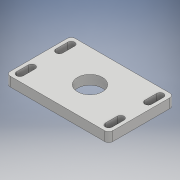
# Autodesk Inventor part: belt tensioner
Saved by Autodesk Inventor 2017 (Build 210142000, 142)
## iProperties
Created: 2018-04-16
Part Number: belt tensioner
Material: Generic
Document SubType Name: Modeling
Designer: RKL
Density: 1 g/cm^3
Appearance: Default
Author: RKL
Autodesk Inventor part; units mm, degrees
ref_plane "YZ Plane" through (0, 0, 0) normal (1, 0, 0) x (0, 1, 0)
ref_plane "XZ Plane" through (0, 0, 0) normal (0, 1, 0) x (-1, 0, 0)
ref_plane "XY Plane" through (0, 0, 0) normal (0, 0, 1) x (1, 0, 0)
sketch "Sketch1" plane through (0, 0, 0) normal (0, 0, 1) x (1, 0, 0)
  line L0 (22.5, -10) -> (-22.5, -10) construction
  line L1 (-22.5, -10) -> (-22.5, 10) construction
  line L2 (-22.5, 10) -> (22.5, 10) construction
  line L3 (22.5, 10) -> (22.5, -10) construction
  line L4 (22.5, -10) -> (-22.5, 10) construction
  line L5 (-22.5, -10) -> (22.5, 10) construction
  line L6 (-22.5, 13) -> (-22.5, 7) construction
  line L7 (-24.25, 13) -> (-24.25, 7)
  line L8 (-20.75, 7) -> (-20.75, 13)
  arc A0 (-20.75, 13) -> (-24.25, 13) centre (-22.5, 13) ccw
  arc A1 (-24.25, 7) -> (-20.75, 7) centre (-22.5, 7) ccw
  line L9 (-22.5, -13) -> (-22.5, -7) construction
  line L10 (-20.75, -13) -> (-20.75, -7)
  line L11 (-24.25, -7) -> (-24.25, -13)
  arc A2 (-24.25, -13) -> (-20.75, -13) centre (-22.5, -13) ccw
  arc A3 (-20.75, -7) -> (-24.25, -7) centre (-22.5, -7) ccw
  line L12 (22.5, 13) -> (22.5, 7) construction
  line L13 (20.75, 13) -> (20.75, 7)
  line L14 (24.25, 7) -> (24.25, 13)
  arc A4 (24.25, 13) -> (20.75, 13) centre (22.5, 13) ccw
  arc A5 (20.75, 7) -> (24.25, 7) centre (22.5, 7) ccw
  line L15 (22.5, -13) -> (22.5, -7) construction
  line L16 (24.25, -13) -> (24.25, -7)
  line L17 (20.75, -7) -> (20.75, -13)
  arc A6 (20.75, -13) -> (24.25, -13) centre (22.5, -13) ccw
  arc A7 (24.25, -7) -> (20.75, -7) centre (22.5, -7) ccw
  line L18 (26, -16.5) -> (-26, -16.5)
  line L19 (-26, -16.5) -> (-26, 16.5)
  line L20 (-26, 16.5) -> (26, 16.5)
  line L21 (26, 16.5) -> (26, -16.5)
  line L22 (26, -16.5) -> (-26, 16.5) construction
  line L23 (-26, -16.5) -> (26, 16.5) construction
  circle A8 centre (0, 0) radius 6.35
  dimension "d0" = 45
  dimension "d1" = 20
  dimension "d2" = 3.5
  dimension "d3" = 6
  dimension "d4" = 52
  dimension "d5" = 33
  dimension "d6" = 12.7
  constraints: 56 end point, 16 point on circle, 16 tangent, 9 centre point, 8 midpoint, 8 parallel, 4 point on line, 3 equal length, 3 equal radius, 2 horizontal, 2 perpendicular, 1 coincident
  measures "d0" distance of L1.end L2.end
  measures "d1" distance of L0.end L1.end
  measures "d2" distance between parallel lines of L8 L7
  measures "d3" distance of L11.start L11.end
  measures "d4" distance of L19.end L20.end
  measures "d5" distance of L18.end L19.end
  measures "d6" diameter of A8
extrude "Extrusion1" add sketch "Sketch1" along normal blind 4.7625
fillet "Fillet1" radius 2 4 edges at (-26, 16.5, 2.3813) (26, 16.5, 2.3813) (26, -16.5, 2.3813) (-26, -16.5, 2.3813)
body "Solid1"
